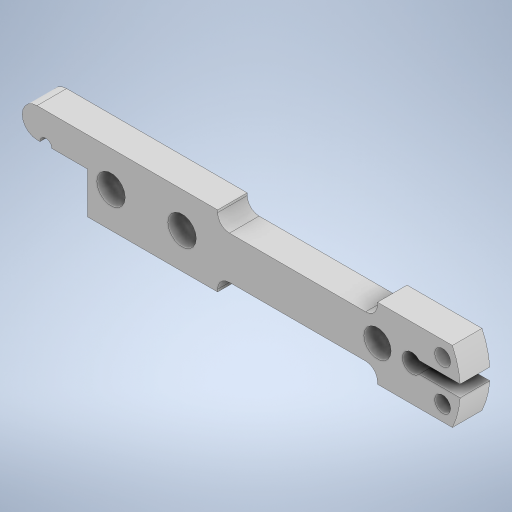
# Autodesk Inventor part: Деталь5
Saved by Autodesk Inventor 2024 (Build 280153000, 153)
## iProperties
Created: 2024-10-31
Part Number: Деталь5
Material: Типовые
Document SubType Name: Modeling
Designer: БАЛАК
Density: 1 g/cm^3
Appearance: По умолчанию
Author: БАЛАК
Autodesk Inventor part; units mm, degrees
ref_plane "YZ Plane" through (0, 0, 0) normal (1, 0, 0) x (0, 1, 0)
ref_plane "XZ Plane" through (0, 0, 0) normal (0, 1, 0) x (-1, 0, 0)
ref_plane "XY Plane" through (0, 0, 0) normal (0, 0, 1) x (1, 0, 0)
sketch "Эскиз1" plane through (0, 0, 0) normal (0, 0, 1) x (1, 0, 0)
  circle A0 centre (0, 12) radius 4.6
  line L0 (0, 24) -> (0, 0)
  arc A1 (25.2982, 0) -> (25.2982, 24) centre (0, 12) ccw
  line L1 (0, 24) -> (25.2982, 24)
  line L2 (14.098, 10) -> (27.9285, 10)
  circle A2 centre (22, 5.2) radius 2.7
  line L3 (0, 0) -> (25.2982, 0)
  circle A3 centre (22, 18.8) radius 2.7
  arc A4 (14.098, 14) -> (14.098, 10) centre (11.6, 12) ccw
  line L4 (14.098, 14) -> (27.9285, 14)
  line L5 (0, 0) -> (0, 0.8)
  line L6 (-4, 4.8) -> (-50, 4.8)
  line L7 (-54, 0.8) -> (-54, 0)
  line L8 (-54, 0) -> (-98, 0)
  arc A5 (-50, 4.8) -> (-54, 0.8) centre (-50, 0.8) ccw
  arc A6 (0, 0.8) -> (-4, 4.8) centre (-4, 0.8) ccw
  line L9 (0, 12) -> (-66, 12)
  circle A7 centre (-66, 12) radius 4.8
  line L10 (-66, 12) -> (-90, 12)
  circle A8 centre (-90, 12) radius 4.8
  line L11 (-4, 19.2) -> (-50, 19.2)
  line L12 (-54, 24) -> (-98, 24)
  arc A9 (-54, 23.2) -> (-50, 19.2) centre (-50, 23.2) ccw
  arc A10 (-4, 19.2) -> (0, 23.2) centre (-4, 23.2) ccw
  line L13 (-54, 24) -> (-54, 23.2)
  line L14 (0, 24) -> (0, 23.2)
  line L15 (-98, 24) -> (-115, 24)
  line L16 (-90, 12) -> (-125.2457, 12)
  line L17 (-98, 0) -> (-98, 14)
  line L18 (-112, 24) -> (-112, 14)
  arc A11 (-115, 24) -> (-115, 14) centre (-115, 19) ccw
  arc A12 (-110, 14) -> (-114, 14) centre (-112, 14) ccw
  line L19 (-115, 14) -> (-114, 14)
  line L20 (-110, 14) -> (-98, 14)
  point P0 (0, 4.8)
  point P1 (-112, 19)
  point P2 (-120, 19)
  point P3 (0, 0.4)
  point P4 (-54, 0.4)
  point P5 (-107.6228, 12)
  dimension "d3" = 9.2
  dimension "d5" = 56
  dimension "d10" = 5.4
  dimension "d12" = 6.4
  dimension "d18" = 4
  dimension "d19" = 4
  dimension "d20" = 66
  dimension "d21" = 9.6
  dimension "d22" = 24
  dimension "d23" = 9.6
  dimension "d25" = 14
  dimension "d28" = 5
  dimension "d30" = 8
  dimension "d31" = 98
  dimension "d32" = 54
  dimension "d33" = 4
  dimension "d34" = 2
  constraints: 42 end point, 18 point on circle, 13 centre point, 8 horizontal, 8 symmetric about line, 7 tangent, 5 point on line, 4 coincident, 4 midpoint, 4 vertical, 3 perpendicular, 1 collinear, 2 other
  measures "d3" diameter of A0
  measures "d5" diameter of A1
  measures "d10" diameter of A2
  measures "d12" diameter of A4
  measures "d18" radius of A5
  measures "d19" radius of A6
  measures "d20" distance of L9.start L9.end
  measures "d21" diameter of A7
  measures "d22" distance of L10.start L10.end
  measures "d23" diameter of A8
  measures "d25" distance of L12.end L18.start
  measures "d28" radius of A11
  measures "d30" distance of point (-112, 19) point (-120, 19)
  measures "d31" horizontal distance of L8.end point (0, 0.4)
  measures "d32" distance of point (0, 0.4) point (-54, 0.4)
  measures "d33" diameter of A12
  measures "d34" distance from line of point (-107.623, 12) L20
extrude "Выдавливание1" add sketch "Эскиз1" along normal blind 10 contours A0 L0 L1 A1 L4 A4 L2 L3 | A0 L9 A7 L10 A8 L16 L17 L20 A12 L18 L15 L12 L13 A9 L11 A10 L0 | L0 A6 L6 A5 L7 L8 L17 L16 A8 L10 A7 L9 A0 | L18 A12 L19 A11 L15
